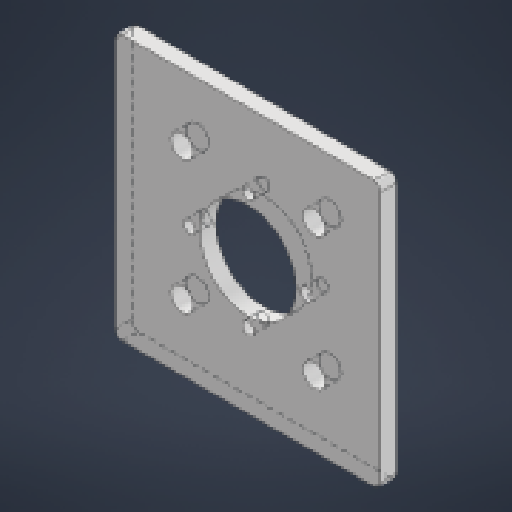
# Autodesk Inventor part: PL_TOP
Saved by Autodesk Inventor 2023 (Build 270158000, 158)
## iProperties
Created: 2025-09-04
Part Number: PL_TOP
Material: 일반
Document SubType Name: Modeling
Designer: k
Density: 1 g/cm^3
Appearance: 기본값
Author: k
Autodesk Inventor part; units mm, degrees
ref_plane "YZ Plane" through (0, 0, 0) normal (1, 0, 0) x (0, 1, 0)
ref_plane "XZ Plane" through (0, 0, 0) normal (0, 1, 0) x (-1, 0, 0)
ref_plane "XY Plane" through (0, 0, 0) normal (0, 0, 1) x (1, 0, 0)
sketch "스케치1" plane through (0, 0, 0) normal (0, 0, 1) x (1, 0, 0)
  line L0 (-49.6566, 38.725) -> (45.3434, 38.725)
  line L1 (47.8434, 36.225) -> (47.8434, -58.775)
  line L2 (45.3434, -61.275) -> (-49.6566, -61.275)
  line L3 (-52.1566, -58.775) -> (-52.1566, 36.225)
  circle A0 centre (-27.1566, 13.725) radius 4.25
  circle A1 centre (22.8434, 13.725) radius 4.25
  circle A2 centre (22.8434, -36.275) radius 4.25
  circle A3 centre (-27.1566, -36.275) radius 4.25
  circle A4 centre (-2.1566, -11.275) radius 22
  circle A5 centre (-2.1566, 10.725) radius 2.25
  circle A6 centre (-24.1566, -11.275) radius 2.25
  circle A7 centre (-2.1566, -33.275) radius 2.25
  circle A8 centre (19.8434, -11.275) radius 2.25
  circle A9 centre (-2.1566, -11.275) radius 18.1
  arc A10 (-49.6566, 38.725) -> (-52.1566, 36.225) centre (-49.6566, 36.225) ccw
  arc A11 (-52.1566, -58.775) -> (-49.6566, -61.275) centre (-49.6566, -58.775) ccw
  arc A12 (45.3434, -61.275) -> (47.8434, -58.775) centre (45.3434, -58.775) ccw
  arc A13 (47.8434, 36.225) -> (45.3434, 38.725) centre (45.3434, 36.225) ccw
  point P0 (0, 0)
  point P1 (-52.1566, 38.725)
  point P2 (47.8434, -61.275)
  point P3 (47.8434, 38.725)
  point P4 (-52.1566, -61.275)
  dimension "d0" = 100
  dimension "d1" = 100
  dimension "d2" = 8.5
  dimension "d3" = 8.5
  dimension "d4" = 8.5
  dimension "d5" = 8.5
  dimension "d6" = 50
  dimension "d7" = 50
  dimension "d8" = 50
  dimension "d9" = 50
  dimension "d10" = 25
  dimension "d11" = 25
  dimension "d12" = 25
  dimension "d13" = 44
  dimension "d14" = 50
  dimension "d15" = 50
  dimension "d16" = 4.5
  dimension "d17" = 4.5
  dimension "d18" = 4.5
  dimension "d19" = 4.5
  dimension "d20" = 36.2
  dimension "d23" = 2.5
  constraints: 14 centre point, 12 point on circle, 8 end point, 8 point on line, 8 tangent, 3 equal radius, 2 parallel, 1 coincident, 1 horizontal, 1 horizontal alignment, 1 perpendicular
  measures "d0" distance of point (47.843, -61.275) point (-52.157, -61.275)
  measures "d1" distance of point (47.843, 38.725) point (47.843, -61.275)
  measures "d2" diameter of A0
  measures "d3" diameter of A1
  measures "d4" diameter of A2
  measures "d5" diameter of A3
  measures "d6" distance of A1.centre A0.centre
  measures "d7" distance of A2.centre A1.centre
  measures "d8" distance of A3.centre A2.centre
  measures "d9" distance of A0.centre A3.centre
  measures "d10" distance from line of L0 A1.centre
  measures "d11" distance from line of L1 A1.centre
  measures "d12" distance from line of L1 A2.centre
  measures "d13" diameter of A4
  measures "d14" distance from line of L0 A4.centre
  measures "d15" distance from line of L3 A4.centre
  measures "d16" diameter of A5
  measures "d17" diameter of A6
  measures "d18" diameter of A7
  measures "d19" diameter of A8
  measures "d20" diameter of A9
  measures "d23" radius of A10
extrude "돌출1" add sketch "스케치1" along normal blind 6 contours L0 A13 L1 A12 L2 A11 L3 A10 | A8 A4 A7 A6 A5
